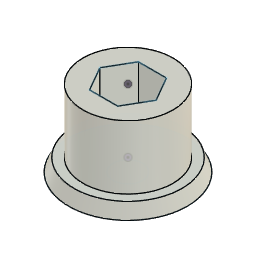
Finneal Mount (Autodesk Fusion 360 design; units mm, degrees)
Autodesk Fusion 360 part; units mm, degrees
sketch "Sketch1" plane through (0, 0, 0) normal (0, 0, 1) x (1, 0, 0)
  circle A0 centre (0, 0) radius 14
  dimension "d1" = 28
  constraint coincident A0.centre origin
  measures "d1" diameter of A0
extrude "Extrude1" add sketch "Sketch1" along normal blind 3 draft -23
sketch "Sketch2" plane through (0, 0, 3) normal (0, 0, 1) x (-1, 0, 0)
  circle A0 centre (0, 0) radius 12.7266
sketch "Sketch3" plane through (0, 0, 3) normal (0, 0, 1) x (-1, 0, 0)
sketch "Sketch4" plane through (0, 0, 3) normal (0, 0, 1) x (-1, 0, 0)
  circle A0 centre (0, 0) radius 10.625
  dimension "d5" = 21.25
  constraint coincident A0.centre origin
  measures "d5" diameter of A0
extrude "Extrude2" add sketch "Sketch4" along normal blind 15
sketch "Sketch5" plane through (0, 0, 18) normal (0, 0, 1) x (-1, 0, 0)
  circle A0 centre (0, 0) radius 10.625
  line L0 (3.3198, -5.75) -> (6.6395, 0)
  line L1 (6.6395, 0) -> (3.3198, 5.75)
  line L2 (3.3198, 5.75) -> (-3.3198, 5.75)
  line L3 (-3.3198, 5.75) -> (-6.6395, 0)
  line L4 (-6.6395, 0) -> (-3.3198, -5.75)
  line L5 (-3.3198, -5.75) -> (3.3198, -5.75)
  dimension "d8" = 5.75
  constraint coincident A0.centre origin
  measures "d8" distance of A0.centre L5
extrude "Extrude3" cut sketch "Sketch5" against normal blind 15 contours L0 L1 L2 L3 L4 L5
hole "Hole1" at (-0.0502, 0.0031, 0) direction (0, 0, 1) diameter 7 depth 3 tip angle 180
sketch "1/4\" Bolt Hole" plane through (0, 0, 0) normal (0, 0, -1) x (1, 0, 0)
  circle A0 centre (-0.0502, -0.0031) radius 3.5
  circle A1 centre (0, 0) radius 14
sketch "Sketch7" plane through (0, 0, 18) normal (0, 0, 1) x (-1, 0, 0)
sketch "Sketch8" plane through (0, 0, 18) normal (0, 0, 1) x (-1, 0, 0)
